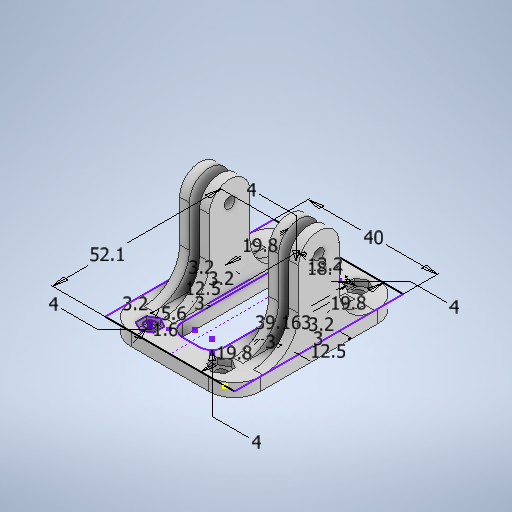
# Autodesk Inventor part: encaixeDuplo2
Saved by Autodesk Inventor 2025 (Build 290162000, 162)
## iProperties
Created: 2024-04-11
Part Number: encaixeDuplo2
Material: Generic
Document SubType Name: Modeling
Designer: cvss2
Density: 1 g/cm^3
Appearance: Default
Author: cvss2
Autodesk Inventor part; units mm, degrees
ref_plane "YZ Plane" through (0, 0, 0) normal (1, 0, 0) x (0, 1, 0)
ref_plane "XZ Plane" through (0, 0, 0) normal (0, 1, 0) x (-1, 0, 0)
ref_plane "XY Plane" through (0, 0, 0) normal (0, 0, 1) x (1, 0, 0)
sketch "Sketch1" plane through (0, 0, 0) normal (0, 1, 0) x (-1, 0, 0)
  circle A0 centre (28, -4.85) radius 1.6
  line L0 (28, -8.0832) -> (25.2, -6.4666)
  line L1 (25.2, -6.4666) -> (25.2, -3.2334)
  line L2 (25.2, -3.2334) -> (28, -1.6168)
  line L3 (28, -1.6168) -> (30.8, -3.2334)
  line L4 (30.8, -3.2334) -> (30.8, -6.4666)
  line L5 (30.8, -6.4666) -> (28, -8.0832)
  line L6 (17, 0) -> (17, -52.1) construction
  line L7 (0, -19.8) -> (0, -32.3)
  line L8 (-3, -52.1) -> (-3, 0)
  line L9 (37, -52.1) -> (37, 0)
  line L10 (-3, -52.1) -> (37, -52.1)
  line L11 (-3, 0) -> (37, 0)
  line L12 (0, -32.3) -> (-3, -32.3)
  line L13 (0, -19.8) -> (-3, -19.8)
  line L14 (3.2, -32.3) -> (3.2, -19.8)
  line L15 (3.2, -19.8) -> (6.2, -19.8)
  line L16 (6.2, -19.8) -> (6.2, -32.3)
  line L17 (6.2, -32.3) -> (3.2, -32.3)
  line L18 (33.8, -32.3) -> (30.8, -32.3)
  line L19 (30.8, -32.3) -> (30.8, -19.8)
  line L20 (30.8, -19.8) -> (33.8, -19.8)
  line L21 (33.8, -19.8) -> (33.8, -32.3)
  line L22 (27.6, -32.3) -> (27.6, -19.8)
  line L23 (27.6, -19.8) -> (24.6, -19.8)
  line L24 (24.6, -19.8) -> (24.6, -32.3)
  line L25 (24.6, -32.3) -> (27.6, -32.3)
  line L26 (9.4, -41.8) -> (24.5, -41.8) construction
  line L27 (10.4, -10.4194) -> (10.4, -41.5824)
  line L28 (14.4, -45.5824) -> (19.6, -45.5824)
  line L29 (23.6, -41.5824) -> (23.6, -10.4194)
  line L30 (19.6, -6.4194) -> (14.4, -6.4194)
  arc A1 (10.4, -41.5824) -> (14.4, -45.5824) centre (14.4, -41.5824) ccw
  arc A2 (14.4, -6.4194) -> (10.4, -10.4194) centre (14.4, -10.4194) ccw
  arc A3 (19.6, -45.5824) -> (23.6, -41.5824) centre (19.6, -41.5824) ccw
  arc A4 (23.6, -10.4194) -> (19.6, -6.4194) centre (19.6, -10.4194) ccw
  point P0 (0, 0)
  point P1 (-1.5, -19.8)
  point P2 (26.1, -19.8)
  point P3 (4.7, -19.8)
  point P4 (32.3, -32.3)
  point P5 (10.4, -6.4194)
  point P6 (10.4, -45.5824)
  point P7 (23.6, -45.5824)
  point P8 (23.6, -6.4194)
  dimension "d2" = 3.2
  dimension "d5" = 5.6
  dimension "d60" = 40
  dimension "d62" = 52.1
  dimension "d63" = 3.2
  dimension "d64" = 3
  dimension "d65" = 3
  dimension "d66" = 3
  dimension "d67" = 12.5
  dimension "d69" = 3.2
  dimension "d70" = 3.2
  dimension "d71" = 12.5
  dimension "d73" = 19.8
  dimension "d74" = 19.8
  dimension "d77" = 19.8
  dimension "d79" = 18.4
  dimension "d85" = 39.163
  dimension "d86" = 13.2
  dimension "d89" = 1.6
  dimension "d111" = 4
  dimension "d112" = 4
  dimension "d113" = 4
  dimension "d114" = 4
  constraints: 62 end point, 17 point on line, 12 perpendicular, 8 point on circle, 8 tangent, 5 centre point, 4 midpoint, 3 horizontal, 3 parallel, 1 coincident, 13 other
  measures "d2" diameter of A0
  measures "d5" distance between parallel lines of L4 L1
  measures "d60" distance between parallel lines of L9 L8
  measures "d62" distance from line of point (0, 0) L10
  measures "d63" distance of L7.end L14.start
  measures "d64" distance of L14.end L15.end
  measures "d65" distance of L22.end L23.end
  measures "d66" distance between parallel lines of L8 L7
  measures "d67" distance from line of point (-1.5, -19.8) L12
  measures "d69" distance between parallel lines of L22 L19
  measures "d70" distance between parallel lines of L9 L21
  measures "d71" distance from line of point (26.1, -19.8) L25
  measures "d73" distance from line of L10 point (32.3, -32.3)
  measures "d74" distance between parallel lines of L10 L12
  measures "d77" distance between parallel lines of L11 L15
  measures "d79" distance between parallel lines of L24 L16
  measures "d85" distance of point (10.4, -6.419) point (10.4, -45.582)
  measures "d86" distance of point (10.4, -45.582) point (23.6, -45.582)
  measures "d89" horizontal distance of point (23.6, -6.419) L0.end
  measures "d111" radius of A1
  measures "d112" radius of A2
  measures "d113" radius of A3
  measures "d114" radius of A4
extrude "Extrusão6" add sketch "Sketch1" against normal blind 4 contours A0 | L0 L1 L2 L3 L4 L5 | L13 L8 L11 L9 L10 L12 L7 | L7 L12 L8 L13 | L14 L15 L16 L17 | L18 L19 L20 L21 | L25 L24 L23 L22 | A2 L30 A4 L29 A3 L28 A1 L27
extrude "Extrusão7" add sketch "Sketch1" along normal blind 30 contours L7 L12 L8 L13 | L14 L15 L16 L17 | L18 L19 L20 L21 | L25 L24 L23 L22
fillet "Arredondamento4" radius 11 8 edges at (1.5, 0, -32.3) (-4.7, 0, -32.3) (-26.1, 0, -32.3) (-32.3, 0, -32.3) (1.5, 0, -19.8) (-4.7, 0, -19.8) (-26.1, 0, -19.8) (-32.3, 0, -19.8)
fillet "Arredondamento5" radius 6.25 8 edges at (1.5, 30, -19.8) (1.5, 30, -32.3) (-4.7, 30, -32.3) (-4.7, 30, -19.8) (-26.1, 30, -19.8) (-26.1, 30, -32.3) (-32.3, 30, -32.3) (-32.3, 30, -19.8)
sketch "Esboço3" plane through (3, -4, 0) normal (1, 0, 0) x (0, 0, -1)
  arc A0 (32.3, 27.75) -> (19.8, 27.75) centre (26.05, 27.75) ccw projected
  circle A1 centre (26.05, 27.75) radius 1.65
  point P0 (0, 4)
  dimension "d96" = 3.3
  constraints: 1 centre point, 1 coincident
  measures "d96" diameter of A1
extrude "Extrusão8" cut sketch "Esboço3" against normal blind 1000
extrude "Extrusão10" cut sketch "Sketch1" against normal blind 1000 contours A0
extrude "Extrusão11" cut sketch "Sketch1" against normal blind 2 contours L0 L1 L2 L3 L4 L5
pattern_linear "Padrão retangular2" count 2 spacing 42.4 along (0, 0, -1) count 2 spacing 22 along (1, 0, 0) of "Extrusão11", "Extrusão10"
extrude "Extrusão12" cut sketch "Sketch1" against normal blind 200 contours A2 L30 A4 L29 A3 L28 A1 L27
fillet "Arredondamento6" radius 8 4 edges at (3, -2, -52.1) (3, -2, 0) (-37, -2, 0) (-37, -2, -52.1)
